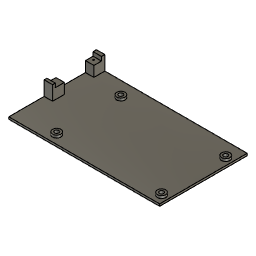
pcb_mount (Autodesk Fusion 360 design; units mm, degrees)
Autodesk Fusion 360 part; units mm, degrees
sketch "boards" plane through (0, 0, 0) normal (0, 0, 1) x (1, 0, 0)
  line L0 (67.31, 49.53) -> (-67.31, 49.53) construction
  line L1 (-67.31, -49.53) -> (67.31, -49.53) construction
  line L2 (67.31, -49.53) -> (67.31, 49.53) construction
  line L3 (67.31, 49.53) -> (-67.31, -49.53) construction
  line L4 (-67.31, 49.53) -> (67.31, -49.53) construction
  circle A0 centre (62.23, 34.29) radius 2.54
  circle A1 centre (62.23, -41.91) radius 2.54
  line L5 (0, 2.5) -> (0, 20)
  circle A2 centre (-62.23, 34.29) radius 2.54
  circle A3 centre (-62.23, -41.91) radius 2.54
  line L6 (-67.31, 49.53) -> (-59.69, 49.53) construction
  line L7 (-59.69, 49.53) -> (-59.69, 44.45) construction
  line L8 (-59.69, 44.45) -> (-59.69, 39.37) construction
  circle A4 centre (-59.69, 39.37) radius 0.5 construction
  circle A5 centre (-59.69, 44.45) radius 0.5 construction
  line L9 (-60.69, 45.45) -> (-58.69, 45.45) construction
  line L10 (-58.69, 45.45) -> (-58.69, 43.45) construction
  line L11 (-58.69, 43.45) -> (-60.69, 43.45) construction
  line L12 (-60.69, 43.45) -> (-60.69, 45.45) construction
  line L13 (-60.69, 45.45) -> (-58.69, 43.45) construction
  line L14 (-58.69, 45.45) -> (-60.69, 43.45) construction
  line L15 (-58.69, 40.37) -> (-60.69, 40.37) construction
  line L16 (-60.69, 40.37) -> (-60.69, 38.37) construction
  line L17 (-60.69, 38.37) -> (-58.69, 38.37) construction
  line L18 (-58.69, 38.37) -> (-58.69, 40.37) construction
  line L19 (-58.69, 40.37) -> (-60.69, 38.37) construction
  line L20 (-60.69, 40.37) -> (-58.69, 38.37) construction
  line L21 (-59.69, 39.37) -> (-59.69, -1.27) construction
  line L22 (-60.69, -0.27) -> (-60.69, -2.27) construction
  line L23 (-60.69, -2.27) -> (-58.69, -2.27) construction
  line L24 (-58.69, -2.27) -> (-58.69, -0.27) construction
  line L25 (-58.69, -0.27) -> (-60.69, -0.27) construction
  circle A6 centre (-59.69, -1.27) radius 0.5 construction
  line L26 (-61.23, 17.51) -> (-63.23, 17.51) construction
  line L27 (-63.23, 17.51) -> (-63.23, 15.51) construction
  line L28 (-63.23, 15.51) -> (-61.23, 15.51) construction
  line L29 (-61.23, 15.51) -> (-61.23, 17.51) construction
  circle A7 centre (-62.23, 16.51) radius 0.5 construction
  line L30 (-59.69, -1.27) -> (-59.69, 16.51) construction
  line L31 (-59.69, 16.51) -> (-62.23, 16.51) construction
  line L32 (-59.69, 49.53) -> (-57.15, 49.53) construction
  line L33 (-59.69, 44.45) -> (-104.862, 44.45) construction
  line L34 (-59.69, 44.45) -> (-59.69, 46.99) construction
  line L35 (-57.15, 46.99) -> (-57.15, 49.53) construction
  line L36 (-57.15, 46.99) -> (-107.15, 46.99)
  line L37 (-107.15, 46.99) -> (-107.15, -6.01)
  line L38 (-107.15, -6.01) -> (-57.15, -6.01)
  line L39 (-57.15, -6.01) -> (-57.15, 46.99)
  circle A8 centre (-104.862, 44.45) radius 0.9
  line L40 (-59.69, -1.27) -> (-59.69, -3.81) construction
  line L41 (-59.69, -3.81) -> (-116, -3.81) construction
  line L42 (-104.862, 44.45) -> (-104.862, -10) construction
  circle A9 centre (-104.862, -3.81) radius 0.9
  point P0 (-59.69, 44.45)
  point P1 (-59.69, 39.37)
  dimension "d1" = 134.62
  dimension "d2" = 99.06
  dimension "d7" = 5.08
  dimension "d8" = 5.08
  dimension "d10" = 5.08
  dimension "d11" = 5.08
  dimension "d18" = 40.64
  dimension "d19" = 17.78
  dimension "d94" = 2.54
  dimension "d95" = 45.172
  dimension "d96" = 2.54
  dimension "d97" = 50
  dimension "d98" = 53
  dimension "d99" = 1.8
  dimension "d100" = 2.54
  dimension "d101" = 1.8
  constraint horizontal L0
  constraint parallel L0 L1
  constraint coincident L3 origin
  constraint coincident L4 origin
  constraint symmetric A0 L5 A2
  constraint symmetric A1 L5 A3
  constraint perpendicular L6 L7
  constraint parallel L7 L8
  constraint coincident P1 L8.end
  constraint coincident P0 L7.end
  constraint horizontal L9
  constraint perpendicular L9 L10
  constraint parallel L9 L11
  constraint parallel L10 L12
  constraint coincident L13 P0
  constraint coincident L14 P0
  constraint horizontal L15
  constraint perpendicular L15 L16
  constraint parallel L15 L17
  constraint parallel L16 L18
  constraint coincident L19 P1
  constraint coincident L20 P1
  constraint perpendicular L17 L21
  constraint horizontal L25
  constraint perpendicular L22 L25
  constraint parallel L23 L25
  constraint parallel L22 L24
  constraint horizontal L26
  constraint perpendicular L26 L27
  constraint parallel L26 L28
  constraint parallel L27 L29
  constraint coincident L21.end A6.centre
  constraint parallel L21 L30
  constraint perpendicular L30 L31
  constraint perpendicular L7 L32
  constraint perpendicular L18 L33
  constraint perpendicular L9 L34
  constraint perpendicular L32 L35
  constraint horizontal L36
  constraint vertical L37
  constraint horizontal L38
  constraint vertical L39
  constraint coincident L33.end A8.centre
  constraint perpendicular L38 L40
  constraint perpendicular L37 L41
  constraint perpendicular L38 L42
  constraint coincident L41 A9.centre
  constraint coincident L42 A9.centre
  measures "d1" distance of L1.start L1.end
  measures "d2" distance of L0.end L1.start
  measures "d7" diameter of A0
  measures "d8" diameter of A1
  measures "d10" distance of L6.end P0
  measures "d11" distance of P0 P1
  measures "d18" distance of P1 L21.end
  measures "d19" distance of L21.end L30.end
  measures "d94" distance of L6.end L32.end
  measures "d95" distance of P0 L33.end
  measures "d96" distance of P0 L34.end
  measures "d97" distance of L35.start L36.end
  measures "d98" distance of L35.start L38.end
  measures "d99" diameter of A8
  measures "d100" distance of L21.end L40.end
  measures "d101" diameter of A9
sketch "mounts" plane through (0, 0, 0) normal (0, 0, 1) x (1, 0, 0)
  circle A0 centre (-62.23, 34.29) radius 2.54
  circle A1 centre (62.23, 34.29) radius 2.54
  circle A2 centre (62.23, -41.91) radius 2.54
  circle A3 centre (-62.23, -41.91) radius 2.54
  circle A4 centre (-62.23, -41.91) radius 5
  circle A5 centre (-62.23, 34.29) radius 5
  circle A6 centre (62.23, 34.29) radius 5
  circle A7 centre (62.23, -41.91) radius 5
  line L0 (-96.21, 44.0508) -> (-98, 44.0508)
  line L1 (70, 52) -> (70, -52)
  line L2 (70, 52) -> (-109, 52)
  line L3 (-109, 52) -> (-109, -52)
  line L4 (-109, 52) -> (-99, 52)
  line L5 (-99, 52) -> (-99, 39)
  line L6 (-99, 39) -> (-109, 39)
  line L7 (-109, 39) -> (-109, 52)
  line L8 (-109, -10) -> (-99, -10)
  line L9 (-99, -10) -> (-99, 4)
  line L10 (-99, 4) -> (-109, 4)
  line L11 (-109, 4) -> (-109, -10)
  line L12 (-99, 48) -> (-109, 48)
  line L13 (-99, -6.7) -> (-109, -6.7)
  circle A8 centre (-104.862, 44.45) radius 0.9
  circle A9 centre (-104.862, -3.81) radius 0.9
  line L14 (70, -52) -> (-109, -52)
  point P0 (-59.69, -1.27)
  dimension "d47" = 10
  dimension "d48" = 10
  dimension "d49" = 10
  dimension "d50" = 10
  constraint concentric A3 A4
  constraint concentric A0 A5
  constraint concentric A1 A6
  constraint concentric A2 A7
  constraint vertical L1
  constraint perpendicular L1 L2
  constraint perpendicular L2 L3
  constraint horizontal L4
  constraint vertical L5
  constraint horizontal L6
  constraint vertical L7
  constraint horizontal L8
  constraint vertical L9
  constraint horizontal L10
  constraint vertical L11
  constraint coincident L3 L8.start
  constraint coincident L5 L12.start
  constraint coincident L7 L12.end
  constraint coincident L9 L13.start
  constraint coincident L11 L13.end
  constraint perpendicular L1 L14
  measures "d47" diameter of A4
  measures "d48" diameter of A5
  measures "d49" diameter of A6
  measures "d50" diameter of A7
extrude "Extrude1" add sketch "mounts" sketch "boards" against normal blind 2.5 contours A4 | A5 | A6 | A7 | L1 L2 L3 L5 L6 L8 L9 L10 L14 | L2 L3 L4 L5 L7 L12 | L3 L5 L6 L7 L12 | L3 L8 L9 L11 L13 | L3 L9 L10 L11 L13 of sketch 2 contours A8 | A9 makes body 1
extrude "Extrude13" add sketch "mounts" along normal blind 3 contours A4 | A5 | A6 | A7 bodies 1
extrude "Extrude4" add sketch "mounts" along normal blind 12.3 contours L3 L5 L6 L7 L12 | L3 L9 L10 L11 L13 bodies 1
extrude "Extrude5" add sketch "mounts" along normal blind 17 contours L2 L3 L4 L5 L7 L12 | L3 L8 L9 L11 L13 bodies 1
sketch "sdcard_mount" plane through (0, 0, 0) normal (0, 0, 1) x (1, 0, 0)
  line L0 (20, 40) -> (38, 40)
  line L1 (38, 40) -> (38, 25)
  line L2 (38, 25) -> (20, 25)
  line L3 (20, 40) -> (38, 40)
  line L4 (38, 40) -> (38, 37)
  line L5 (38, 37) -> (20, 37)
  line L6 (20, 37) -> (38, 37)
  line L7 (38, 37) -> (38, 32)
  line L8 (38, 32) -> (20, 32)
  line L9 (21, 41) -> (21, 37)
  line L10 (37, 41) -> (37, 37)
  circle A0 centre (22, 35) radius 1
  circle A1 centre (36, 35) radius 1
  circle A2 centre (29, 28.6038) radius 1
  line L11 (23.7, 41) -> (23.7, 32)
  line L12 (34.2, 40.5) -> (34.2, 32)
  line L13 (37, 37) -> (37, 25)
  line L14 (21, 37) -> (21, 25)
  line L15 (22, 41) -> (22, 32)
  line L16 (20, 40) -> (19, 40)
  line L17 (19, 40) -> (19, 25)
  line L18 (19, 25) -> (20, 25)
  line L19 (21, 37) -> (19, 37)
  dimension "d79" = 18
  dimension "d80" = 15
  dimension "d81" = 3
  dimension "d82" = 5
  dimension "d83" = 2
  dimension "d84" = 2
  dimension "d85" = 2
  constraint horizontal L0
  constraint vertical L1
  constraint horizontal L2
  constraint horizontal L3
  constraint vertical L4
  constraint horizontal L5
  constraint horizontal L6
  constraint vertical L7
  constraint horizontal L8
  constraint coincident L5 L9.end
  constraint perpendicular L5 L9
  constraint coincident L6 L10.end
  constraint perpendicular L6 L10
  constraint coincident L8 L11.end
  constraint perpendicular L8 L11
  constraint coincident L8 L12.end
  constraint perpendicular L8 L12
  constraint coincident L2 L13.end
  constraint perpendicular L2 L13
  constraint coincident L2 L14.end
  constraint perpendicular L2 L14
  constraint coincident L8 L15.end
  constraint perpendicular L8 L15
  constraint horizontal L16
  constraint vertical L17
  constraint horizontal L18
  constraint coincident L17 L19.end
  constraint perpendicular L17 L19
  measures "d79" distance of L0.start L0.end
  measures "d80" distance of L0.start L2.end
  measures "d81" distance of L0.start L5.end
  measures "d82" distance of L5.end L8.end
  measures "d83" diameter of A0
  measures "d84" diameter of A1
  measures "d85" diameter of A2
extrude "Extrude9" add sketch "sdcard_mount" along normal blind 11 separate body contours L2 L5 L6 L14 L17 L18 L19 | L5 L6 A0 L14 L15 | L5 L6 L8 A0 L11 L15 | L8 A0 L14 L15 | L5 L6 L8 L12 L13 | L1 L5 L6 L7 L8 L13 | L1 L2 L8 L13 makes body 2 at (19, 33, 3.6667) makes body 3 at (38, 33, 3.6667)
extrude "Extrude10" add sketch "sdcard_mount" along normal blind 8.5 contours L2 L8 L13 L14 bodies 2 3
extrude "Extrude11" add sketch "sdcard_mount" along normal blind 9 contours L5 L6 L8 L11 L12 bodies 2
extrude "Extrude12" cut sketch "sdcard_mount" along normal blind 7 contours L5 L6 L8 A0 L11 L15 | L5 L6 L8 L11 L12 bodies 2
hidden bodies 2
named bodies: "board_mount", "sdcard mount"
